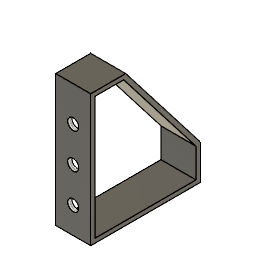
Triangle Bracket (Autodesk Fusion 360 design; units mm, degrees)
Autodesk Fusion 360 part; units mm, degrees
sketch "Sketch1" plane through (0, 0, 0) normal (1, 0, 0) x (0, 1, 0)
  line L0 (0, 0) -> (0, 30)
  line L1 (0, 0) -> (25, 0)
  line L2 (25, 0) -> (25, 8)
  line L3 (0, 30) -> (8, 30)
  line L4 (8, 30) -> (25, 8)
  line L5 (24, 1) -> (24, 7.6587)
  line L6 (7.509, 29) -> (24, 7.6587)
  line L7 (1, 29) -> (7.509, 29)
  line L8 (1, 1) -> (1, 29)
  line L9 (1, 1) -> (24, 1)
  dimension "d1" = 30
  dimension "d2" = 25
  dimension "d3" = 8
  dimension "d4" = 8
  dimension "d5" = 1
  constraint coincident L0.start L1.start
  constraint vertical L0
  constraint perpendicular L0 L1
  constraint perpendicular L1 L2
  constraint perpendicular L0 L3
  measures "d1" distance of L0.start L0.end
  measures "d2" distance of L0.start L1.end
  measures "d3" distance of L1.end L2.end
  measures "d4" distance of L0.end L3.end
extrude "Extrude1" add sketch "Sketch1" along normal mid plane 8
sketch "Sketch2" plane through (0, 0, 0) normal (0, -1, 0) x (1, 0, 0)
  line L0 (-4, 0) -> (4, 0)
  line L1 (4, 0) -> (4, 30)
  line L2 (4, 30) -> (-4, 30)
  line L3 (-4, 30) -> (-4, 0)
  point P0 (0, 6)
  point P1 (0, 14)
  point P2 (0, 22)
  dimension "d8" = 6
  dimension "d9" = 8
  dimension "d10" = 8
  measures "d8" distance of L0 P0
  measures "d9" distance of P0 P1
  measures "d10" distance of P1 P2
hole "Hole1" at (0, 0, 22) at (0, 0, 14) at (0, 0, 6) direction (0, 1, 0) diameter 2.529 depth 8 tip angle 118
thread "Thread1" "ISO Metric profile 3.0 M3x0.5 M3x0.5 6H" thread offset 0 thread depth 7.4
